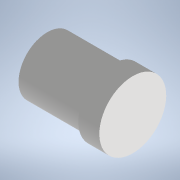
# Autodesk Inventor part: 00_cctvlens
Saved by Autodesk Inventor 2022 (Build 260153000, 153)
## iProperties
Created: 2022-06-11
Part Number: 00_cctvlens
Material: Generisch
Document SubType Name: Modeling
Designer: diederichbenedict
Density: 1 g/cm^3
Appearance: Vorgabe
Author: diederichbenedict
Autodesk Inventor part; units mm, degrees
ref_plane "YZ Plane" through (0, 0, 0) normal (1, 0, 0) x (0, 1, 0)
ref_plane "XZ Plane" through (0, 0, 0) normal (0, 1, 0) x (-1, 0, 0)
ref_plane "XY Plane" through (0, 0, 0) normal (0, 0, 1) x (1, 0, 0)
sketch "Skizze1" plane through (0, 0, 0) normal (0, 0, 1) x (1, 0, 0)
  line L0 (0, 0) -> (0, 6)
  line L1 (0, 6) -> (13.5, 6)
  line L2 (13.5, 6) -> (13.5, 7)
  line L3 (13.5, 7) -> (17.9, 7)
  line L4 (17.9, 7) -> (17.9, 0)
  line L5 (17.9, 0) -> (0, 0)
  dimension "d0" = 6
  dimension "d1" = 13.5
  dimension "d2" = 7
  dimension "d3" = 4.4
  constraints: 12 end point, 5 perpendicular, 1 vertical
  measures "d0" distance of L0.start L0.end
  measures "d1" distance of L0.end L1.end
  measures "d2" distance between parallel lines of L5 L3
  measures "d3" distance from line of L2.end L4
revolve "Umdrehung1" add sketch "Skizze1" angle 360 about axis through (17.9, 0, 0) along (-1, 0, 0)
